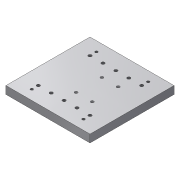
# Autodesk Inventor part: Befestigungsplatte
Saved by Autodesk Inventor 2016 (Build 200138000, 138)
## iProperties
Created: 2015-07-27
Part Number: Befestigungsplatte
Material: Aluminum 6061
Document SubType Name: Modeling
Density: 2.7 g/cm^3
Appearance: Aluminum - Flat
Mass: 684.45 g
Surface Area: 416 cm^2
Volume: 253.5 cm^3
Autodesk Inventor part; units mm, degrees
ref_plane "YZ Plane" through (0, 0, 0) normal (1, 0, 0) x (0, 1, 0)
ref_plane "XZ Plane" through (0, 0, 0) normal (0, 1, 0) x (-1, 0, 0)
ref_plane "XY Plane" through (0, 0, 0) normal (0, 0, 1) x (1, 0, 0)
sketch "Sketch1" plane through (0, 0, 0) normal (0, 0, 1) x (1, 0, 0)
  line L0 (-65, -65) -> (65, -65)
  line L1 (65, -65) -> (65, 65)
  line L2 (65, 65) -> (-65, 65)
  line L3 (-65, 65) -> (-65, -65)
  line L4 (-65, -65) -> (65, 65) construction
  line L5 (65, -65) -> (-65, 65) construction
  point P0 (0, 0)
  dimension "d0" = 130
  dimension "d1" = 130
  constraints: 12 end point, 2 midpoint, 2 parallel, 1 horizontal, 1 perpendicular
  measures "d0" distance of L2.end L1.end
  measures "d1" distance of L1.end L0.end
extrude "Extrusion1" add sketch "Sketch1" along normal blind 12
sketch "Sketch2" plane through (0, 0, 12) normal (0, 0, 1) x (1, 0, 0)
  line L0 (-65, -65) -> (65, -65) projected
  line L1 (65, -65) -> (65, 65) projected
  line L2 (65, 65) -> (-65, 65) projected
  point P0 (0, 0)
  point P1 (40, -40)
  point P2 (40, 40)
  point P3 (0, 40)
  point P4 (-40, 40)
  point P5 (-40, -40)
  point P6 (0, -40)
  dimension "d4" = 40
  dimension "d5" = 40
  dimension "d7" = 25
  dimension "d8" = 25
  dimension "d9" = 25
  constraints: 4 horizontal alignment, 3 vertical alignment
  measures "d4" distance of point (0, -40) point (40, -40)
  measures "d5" distance of point (-40, -40) point (0, -40)
  measures "d7" distance from line of L0 point (40, -40)
  measures "d8" distance from line of L1 point (40, -40)
  measures "d9" distance from line of L2 point (40, 40)
hole "Hole1" at (40, -40, 12) at (40, 40, 12) at (0, 40, 12) at (-40, 40, 12) at (-40, -40, 12) at (0, -40, 12) direction (0, 0, -1) diameter 4.917 end through all thread size "M6x1" designation "M6" class "6H" standard "ISO Metric profile"
sketch "Sketch3" plane through (0, 0, 12) normal (0, 0, 1) x (1, 0, 0)
  line L0 (-1.5, 20) -> (23.5, 20)
  line L1 (23.5, 20) -> (23.5, -20)
  line L2 (23.5, -20) -> (-1.5, -20)
  line L3 (-1.5, -20) -> (-1.5, 20)
  line L4 (65, -65) -> (65, 65) projected
  point P0 (0, 0)
  point P1 (-1.5, 0)
  dimension "d17" = 40
  dimension "d18" = 25
  dimension "d19" = 41.5
  constraints: 8 end point, 2 parallel, 1 horizontal, 1 horizontal alignment, 1 midpoint, 1 perpendicular
  measures "d17" distance of L0.end L1.end
  measures "d18" distance of L0.start L0.end
  measures "d19" distance between parallel lines of L4 L1
hole "Hole2" at (23.5, 20, 12) at (-1.5, 20, 12) at (-1.5, -20, 12) at (23.5, -20, 12) direction (0, 0, -1) diameter 4.5 end through all clearance for "Socket Head Cap Screw ISO 4762" size "M4" standard "ISO"
sketch "Sketch4" plane through (0, 0, 12) normal (0, 0, 1) x (1, 0, 0)
  line L0 (-20, 40) -> (20, 40)
  line L1 (20, 40) -> (20, -40)
  line L2 (20, -40) -> (-20, -40)
  line L3 (-20, -40) -> (-20, 40)
  circle A0 centre (40, -40) radius 2.4585 projected
  circle A1 centre (0, -40) radius 2.4585 projected
  circle A2 centre (0, 40) radius 2.4585 projected
  point P0 (0, 0)
  dimension "d27" = 40
  dimension "d28" = 20
  constraints: 8 end point, 2 midpoint, 2 parallel, 1 horizontal, 1 perpendicular
  measures "d27" distance of L1.end L2.end
  measures "d28" distance from line of A0.centre L1
hole "Hole3" at (20, -40, 12) at (-20, -40, 12) at (-20, 40, 12) at (20, 40, 12) direction (0, 0, -1) diameter 4.917 end through all thread size "M6x1" designation "M6" class "6H" standard "ISO Metric profile"
sketch "Sketch5" plane through (0, 0, 0) normal (0, 0, -1) x (-1, 0, 0)
  line L0 (40, -50) -> (-40, -50)
  line L1 (-40, -50) -> (-40, 50)
  line L2 (-40, 50) -> (40, 50)
  line L3 (40, 50) -> (40, -50)
  line L4 (-65, -65) -> (-65, 65) projected
  line L5 (-65, 65) -> (65, 65) projected
  line L6 (65, -65) -> (-65, -65) projected
  line L7 (65, 65) -> (65, -65) projected
  point P0 (0, 0)
  dimension "d36" = 25
  dimension "d38" = 15
  dimension "d39" = 15
  dimension "d40" = 25
  constraints: 8 end point, 2 parallel, 1 horizontal, 1 perpendicular
  measures "d36" distance between parallel lines of L4 L1
  measures "d38" distance between parallel lines of L5 L2
  measures "d39" distance between parallel lines of L6 L0
  measures "d40" distance between parallel lines of L7 L3
hole "Hole4" at (-40, -50, 0) at (40, -50, 0) at (40, 50, 0) at (-40, 50, 0) direction (0, 0, 1) diameter 4.134 end through all thread size "M5x0.8" designation "M5" class "6H" standard "ISO Metric profile"
equation "\"d9\" = d7"
equation "\"d28\" = 0.5 * d27"
equation "\"d39\" = d38"
equation "\"d40\" = d36"
body "Solid1"
